Autodesk Inventor part; units mm, degrees
(part 3 of 3)
sketch "Sketch1 outline for Extrusion18" plane through (0, 0, 0) normal (1, 0, 0) x (0, 1, 0)
  line L0 (33.007036, -41.557309) -> (32.83808, -40.490169)
  line L1 (32.83808, -40.490169) -> (32.684563, -39.64781)
  line L2 (32.684563, -39.64781) -> (32.342536, -38.633206)
  line L3 (32.342536, -38.633206) -> (31.917915, -37.441578)
  line L4 (31.917915, -37.441578) -> (31.333308, -36.42555)
  line L5 (31.333308, -36.42555) -> (30.795289, -35.506434)
  line L6 (30.795289, -35.506434) -> (29.641867, -34.174329)
  line L7 (29.641867, -34.174329) -> (29.315032, -33.800203)
  line L8 (29.315032, -33.800203) -> (27.540481, -32.409054)
  line L9 (27.540481, -32.409054) -> (27.014126, -32.133714)
  line L10 (27.014126, -32.133714) -> (25.524659, -31.369786)
  line L11 (25.524659, -31.369786) -> (24.698398, -31.122197)
  line L12 (24.698398, -31.122197) -> (23.29583, -30.72275)
  line L13 (23.29583, -30.72275) -> (22.602461, -30.632692)
  line L14 (22.602461, -30.632692) -> (21.504026, -30.512373)
  line L15 (21.504026, -30.512373) -> (21.030936, -30.512373)
  line L16 (21.030936, -30.512373) -> (20.906647, -30.514104)
  line L17 (20.906647, -30.514104) -> (20.804876, -30.516691)
  line L18 (20.804876, -30.516691) -> (20.202896, -30.530407)
  line L19 (20.202896, -30.530407) -> (18.407116, -30.815395)
  line L20 (18.407116, -30.815395) -> (16.184616, -31.565203)
  line L21 (16.184616, -31.565203) -> (14.183096, -32.714553)
  line L22 (14.183096, -32.714553) -> (12.450816, -34.213661)
  line L23 (12.450816, -34.213661) -> (11.036036, -36.015029)
  line L24 (11.036036, -36.015029) -> (9.984476, -38.066841)
  line L25 (9.984476, -38.066841) -> (9.346936, -40.324139)
  line L26 (9.346936, -40.324139) -> (9.146306, -42.133114)
  line L27 (9.146306, -42.133114) -> (9.164056, -42.734345)
  line L28 (9.164056, -42.734345) -> (9.174216, -43.325403)
  line L29 (9.174216, -43.325403) -> (9.453616, -45.097561)
  line L30 (9.453616, -45.097561) -> (9.822098, -46.206473)
  line L31 (9.822098, -46.206473) -> (10.19878, -47.320103)
  line L32 (10.19878, -47.320103) -> (10.628979, -48.084172)
  line L33 (10.628979, -48.084172) -> (11.336866, -49.317963)
  line L34 (11.336866, -49.317963) -> (11.882186, -49.960017)
  line L35 (11.882186, -49.960017) -> (12.817178, -51.038904)
  line L36 (12.817178, -51.038904) -> (13.54104, -51.62178)
  line L37 (13.54104, -51.62178) -> (14.594831, -52.448813)
  line L38 (14.594831, -52.448813) -> (15.440099, -52.899261)
  line L39 (15.440099, -52.899261) -> (16.628337, -53.507219)
  line L40 (16.628337, -53.507219) -> (17.574428, -53.796043)
  line L41 (17.574428, -53.796043) -> (18.877281, -54.167378)
  line L42 (18.877281, -54.167378) -> (19.560515, -54.257796)
  line L43 (19.560515, -54.257796) -> (20.689085, -54.381464)
  line L44 (20.689085, -54.381464) -> (21.150316, -54.381464)
  line L45 (21.150316, -54.381464) -> (21.356056, -54.377324)
  line L46 (21.356056, -54.377324) -> (21.378916, -54.377324)
  line L47 (21.378916, -54.377324) -> (21.979406, -54.361994)
  line L48 (21.979406, -54.361994) -> (22.13415, -54.337482)
  line L49 (22.13415, -54.337482) -> (24.575291, -53.808384)
  line L50 (24.575291, -53.808384) -> (25.423153, -53.522407)
  line L51 (25.423153, -53.522407) -> (27.202918, -52.636602)
  line L52 (27.202918, -52.636602) -> (27.998156, -52.179361)
  line L53 (27.998156, -52.179361) -> (29.730436, -50.679973)
  line L54 (29.730436, -50.679973) -> (31.145216, -48.878859)
  line L55 (31.145216, -48.878859) -> (32.196776, -46.825777)
  line L56 (32.196776, -46.825777) -> (32.836856, -44.569749)
  line L57 (32.836856, -44.569749) -> (33.034976, -42.760507)
  line L58 (33.034976, -42.760507) -> (33.022276, -42.159543)
  line L59 (33.022276, -42.159543) -> (33.007036, -41.557309)
  line L60 (-22.169384, -48.611651) -> (-23.518124, -50.252745)
  line L61 (-23.518124, -50.252745) -> (-24.111863, -51.312447)
  line L62 (-24.111863, -51.312447) -> (-24.588154, -52.192295)
  line L63 (-24.588154, -52.192295) -> (-24.905044, -53.119435)
  line L64 (-24.905044, -53.119435) -> (-25.301336, -54.389917)
  line L65 (-25.301336, -54.389917) -> (-25.419783, -55.059031)
  line L66 (-25.419783, -55.059031) -> (-25.56963, -56.17919)
  line L67 (-25.56963, -56.17919) -> (-25.578064, -56.345164)
  line L68 (-25.578064, -56.345164) -> (-25.593304, -56.661836)
  line L69 (-25.593304, -56.661836) -> (-25.593304, -57.024666)
  line L70 (-25.593304, -57.024666) -> (-25.521621, -58.095078)
  line L71 (-25.521621, -58.095078) -> (-25.430368, -58.777249)
  line L72 (-25.430368, -58.777249) -> (-25.204455, -59.836085)
  line L73 (-25.204455, -59.836085) -> (-24.794771, -61.149472)
  line L74 (-24.794771, -61.149472) -> (-24.482688, -61.917917)
  line L75 (-24.482688, -61.917917) -> (-23.833695, -63.116856)
  line L76 (-23.833695, -63.116856) -> (-23.403552, -63.814127)
  line L77 (-23.403552, -63.814127) -> (-22.425656, -64.997007)
  line L78 (-22.425656, -64.997007) -> (-22.021991, -65.457083)
  line L79 (-22.021991, -65.457083) -> (-20.383214, -66.812521)
  line L80 (-20.383214, -66.812521) -> (-19.879408, -67.099838)
  line L81 (-19.879408, -67.099838) -> (-18.440429, -67.879534)
  line L82 (-18.440429, -67.879534) -> (-18.074437, -68.024885)
  line L83 (-18.074437, -68.024885) -> (-16.530305, -68.504563)
  line L84 (-16.530305, -68.504563) -> (-15.016744, -68.589031)
  line L85 (-15.016744, -68.589031) -> (-14.849104, -68.58489)
  line L86 (-14.849104, -68.58489) -> (-14.452864, -68.571098)
  line L87 (-14.452864, -68.571098) -> (-10.625084, -68.415371)
  line L88 (-10.625084, -68.415371) -> (-10.477781, -68.408219)
  line L89 (-10.477781, -68.408219) -> (-9.069068, -67.970607)
  line L90 (-9.069068, -67.970607) -> (-6.901029, -66.782518)
  line L91 (-6.901029, -66.782518) -> (-6.724497, -66.636927)
  line L92 (-6.724497, -66.636927) -> (-4.410069, -64.414728)
  line L93 (-4.410069, -64.414728) -> (-4.038829, -63.964888)
  line L94 (-4.038829, -63.964888) -> (-2.494622, -61.063215)
  line L95 (-2.494622, -61.063215) -> (-2.230518, -60.213444)
  line L96 (-2.230518, -60.213444) -> (-1.848254, -58.490356)
  line L97 (-1.848254, -58.490356) -> (-1.722384, -57.559208)
  line L98 (-1.722384, -57.559208) -> (-1.722384, -56.356162)
  line L99 (-1.722384, -56.356162) -> (-1.79223, -55.839475)
  line L100 (-1.79223, -55.839475) -> (-1.982369, -54.500406)
  line L101 (-1.982369, -54.500406) -> (-2.17304, -53.8869)
  line L102 (-2.17304, -53.8869) -> (-2.717481, -52.211101)
  line L103 (-2.717481, -52.211101) -> (-3.113204, -51.481774)
  line L104 (-3.113204, -51.481774) -> (-3.865434, -50.160677)
  line L105 (-3.865434, -50.160677) -> (-4.4666, -49.432156)
  line L106 (-4.4666, -49.432156) -> (-5.380475, -48.386819)
  line L107 (-5.380475, -48.386819) -> (-6.157427, -47.746057)
  line L108 (-6.157427, -47.746057) -> (-7.207823, -46.941879)
  line L109 (-7.207823, -46.941879) -> (-8.154694, -46.428219)
  line L110 (-8.154694, -46.428219) -> (-9.292197, -45.87547)
  line L111 (-9.292197, -45.87547) -> (-10.362386, -45.543008)
  line L112 (-10.362386, -45.543008) -> (-11.715458, -45.204164)
  line L113 (-11.715458, -45.204164) -> (-12.392664, -45.113647)
  line L114 (-12.392664, -45.113647) -> (-13.657176, -45.024663)
  line L115 (-13.657176, -45.024663) -> (-14.090958, -45.024663)
  line L116 (-14.090958, -45.024663) -> (-14.451188, -45.049937)
  line L117 (-14.451188, -45.049937) -> (-15.697902, -45.216811)
  line L118 (-15.697902, -45.216811) -> (-16.261766, -45.327388)
  line L119 (-16.261766, -45.327388) -> (-17.578172, -45.736339)
  line L120 (-17.578172, -45.736339) -> (-18.526645, -46.082568)
  line L121 (-18.526645, -46.082568) -> (-19.456689, -46.586467)
  line L122 (-19.456689, -46.586467) -> (-20.493311, -47.193856)
  line L123 (-20.493311, -47.193856) -> (-21.065728, -47.667296)
  line L124 (-21.065728, -47.667296) -> (-22.169384, -48.611651)
  line L125 (-52.369984, -60.267051) -> (-49.128944, -61.227526)
  line L126 (-55.415444, -58.665759) -> (-52.369984, -60.267051)
  line L127 (-57.536344, -57.046585) -> (-55.415444, -58.665759)
  line L128 (-58.158644, -56.423701) -> (-57.536344, -57.046585)
  line L129 (-58.783484, -55.799445) -> (-58.158644, -56.423701)
  line L130 (-60.404004, -53.677275) -> (-58.783484, -55.799445)
  line L131 (-62.004204, -50.634507) -> (-60.404004, -53.677275)
  line L132 (-62.964324, -47.390673) -> (-62.004204, -50.634507)
  line L133 (-63.286904, -44.048795) -> (-62.964324, -47.390673)
  line L134 (-62.964324, -40.705901) -> (-63.286904, -44.048795)
  line L135 (-62.004204, -37.463337) -> (-62.964324, -40.705901)
  line L136 (-60.404004, -34.419147) -> (-62.004204, -37.463337)
  line L137 (-58.783484, -32.297231) -> (-60.404004, -34.419147)
  line L138 (-58.158644, -31.674169) -> (-58.783484, -32.297231)
  line L139 (-57.536344, -31.049837) -> (-58.158644, -31.674169)
  line L140 (-55.415444, -29.430841) -> (-57.536344, -31.049837)
  line L141 (-52.369984, -27.829625) -> (-55.415444, -29.430841)
  line L142 (-49.128944, -26.868997) -> (-52.369984, -27.829625)
  line L143 (-45.786304, -26.547941) -> (-49.128944, -26.868997)
  line L144 (-42.443664, -26.868997) -> (-45.786304, -26.547941)
  line L145 (-39.200084, -27.829625) -> (-42.443664, -26.868997)
  line L146 (-36.157164, -29.430841) -> (-39.200084, -27.829625)
  line L147 (-34.033724, -31.049837) -> (-36.157164, -29.430841)
  line L148 (-33.408884, -31.674169) -> (-34.033724, -31.049837)
  line L149 (-32.789124, -32.297231) -> (-33.408884, -31.674169)
  line L150 (-31.168604, -34.419147) -> (-32.789124, -32.297231)
  line L151 (-29.568404, -37.463337) -> (-31.168604, -34.419147)
  line L152 (-28.605744, -40.705901) -> (-29.568404, -37.463337)
  line L153 (-28.283164, -44.048795) -> (-28.605744, -40.705901)
  line L154 (-28.605744, -47.390673) -> (-28.283164, -44.048795)
  line L155 (-29.568404, -50.634507) -> (-28.605744, -47.390673)
  line L156 (-31.168604, -53.677275) -> (-29.568404, -50.634507)
  line L157 (-32.789124, -55.799445) -> (-31.168604, -53.677275)
  line L158 (-33.408884, -56.423701) -> (-32.789124, -55.799445)
  line L159 (-34.033724, -57.046585) -> (-33.408884, -56.423701)
  line L160 (-36.157164, -58.665759) -> (-34.033724, -57.046585)
  line L161 (-39.200084, -60.267051) -> (-36.157164, -58.665759)
  line L162 (-42.443664, -61.227526) -> (-39.200084, -60.267051)
  line L163 (-45.786304, -61.548633) -> (-42.443664, -61.227526)
  line L164 (-49.128944, -61.227526) -> (-45.786304, -61.548633)
  line L165 (-59.479444, 24.131155) -> (-60.083964, 21.865475)
  line L166 (-60.083964, 21.865475) -> (-60.199445, 20.635684)
  line L167 (-60.199445, 20.635684) -> (-60.235804, 19.618519)
  line L168 (-60.235804, 19.618519) -> (-60.228744, 19.451205)
  line L169 (-60.228744, 19.451205) -> (-60.205884, 18.851765)
  line L170 (-60.205884, 18.851765) -> (-59.895339, 17.084166)
  line L171 (-59.895339, 17.084166) -> (-59.690576, 16.492921)
  line L172 (-59.690576, 16.492921) -> (-59.126949, 14.900308)
  line L173 (-59.126949, 14.900308) -> (-58.65977, 14.095394)
  line L174 (-58.65977, 14.095394) -> (-57.971801, 12.941087)
  line L175 (-57.971801, 12.941087) -> (-57.323583, 12.191296)
  line L176 (-57.323583, 12.191296) -> (-56.476925, 11.244335)
  line L177 (-56.476925, 11.244335) -> (-55.678233, 10.610482)
  line L178 (-55.678233, 10.610482) -> (-54.690294, 9.860171)
  line L179 (-54.690294, 9.860171) -> (-53.784254, 9.384239)
  line L180 (-53.784254, 9.384239) -> (-52.659665, 8.831052)
  line L181 (-52.659665, 8.831052) -> (-51.657409, 8.529209)
  line L182 (-51.657409, 8.529209) -> (-50.388844, 8.190593)
  line L183 (-50.388844, 8.190593) -> (-49.709686, 8.101058)
  line L184 (-49.709686, 8.101058) -> (-48.575756, 7.994027)
  line L185 (-48.575756, 7.994027) -> (-48.224704, 7.994027)
  line L186 (-48.224704, 7.994027) -> (-47.958004, 7.999615)
  line L187 (-47.958004, 7.999615) -> (-47.938503, 7.999615)
  line L188 (-47.938503, 7.999615) -> (-47.828464, 8.003933)
  line L189 (-47.828464, 8.003933) -> (-47.350022, 8.023598)
  line L190 (-47.350022, 8.023598) -> (-46.652701, 8.12955)
  line L191 (-46.652701, 8.12955) -> (-45.680707, 8.299855)
  line L192 (-45.680707, 8.299855) -> (-44.809198, 8.564772)
  line L193 (-44.809198, 8.564772) -> (-43.526766, 9.019144)
  line L194 (-43.526766, 9.019144) -> (-42.720858, 9.425909)
  line L195 (-42.720858, 9.425909) -> (-41.579317, 10.105711)
  line L196 (-41.579317, 10.105711) -> (-40.934583, 10.582054)
  line L197 (-40.934583, 10.582054) -> (-39.793143, 11.604587)
  line L198 (-39.793143, 11.604587) -> (-39.40199, 12.011768)
  line L199 (-39.40199, 12.011768) -> (-38.289337, 13.473296)
  line L200 (-38.289337, 13.473296) -> (-38.109165, 13.74007)
  line L201 (-38.109165, 13.74007) -> (-37.16308, 15.662676)
  line L202 (-37.16308, 15.662676) -> (-37.127948, 15.741932)
  line L203 (-37.127948, 15.741932) -> (-36.528004, 17.991721)
  line L204 (-36.528004, 17.991721) -> (-36.407377, 19.257413)
  line L205 (-36.407377, 19.257413) -> (-36.383619, 20.472644)
  line L206 (-36.383619, 20.472644) -> (-36.384985, 20.504957)
  line L207 (-36.384985, 20.504957) -> (-36.715964, 22.778859)
  line L208 (-36.715964, 22.778859) -> (-36.898866, 23.305176)
  line L209 (-36.898866, 23.305176) -> (-37.482851, 24.950917)
  line L210 (-37.482851, 24.950917) -> (-37.922645, 25.712215)
  line L211 (-37.922645, 25.712215) -> (-38.623993, 26.888971)
  line L212 (-38.623993, 26.888971) -> (-39.285921, 27.663664)
  line L213 (-39.285921, 27.663664) -> (-40.093943, 28.56811)
  line L214 (-40.093943, 28.56811) -> (-40.939105, 29.251808)
  line L215 (-40.939105, 29.251808) -> (-41.847578, 29.942526)
  line L216 (-41.847578, 29.942526) -> (-42.823468, 30.47202)
  line L217 (-42.823468, 30.47202) -> (-43.908, 31.00537)
  line L218 (-43.908, 31.00537) -> (-44.404458, 31.181517)
  line L219 (-44.404458, 31.181517) -> (-46.370504, 31.705943)
  line L220 (-46.370504, 31.705943) -> (-48.181524, 31.876885)
  line L221 (-48.181524, 31.876885) -> (-48.780964, 31.851993)
  line L222 (-48.780964, 31.851993) -> (-49.380404, 31.828625)
  line L223 (-49.380404, 31.828625) -> (-51.173644, 31.514427)
  line L224 (-51.173644, 31.514427) -> (-53.383444, 30.730583)
  line L225 (-53.383444, 30.730583) -> (-55.367184, 29.550753)
  line L226 (-55.367184, 29.550753) -> (-57.074064, 28.023959)
  line L227 (-57.074064, 28.023959) -> (-58.458364, 26.200747)
  line L228 (-58.458364, 26.200747) -> (-59.479444, 24.131155)
  line L229 (-9.649724, 33.651837) -> (-11.958584, 33.632533)
  line L230 (-7.345944, 33.213687) -> (-9.649724, 33.651837)
  line L231 (-5.639064, 32.579703) -> (-7.345944, 33.213687)
  line L232 (-5.105664, 32.297255) -> (-5.639064, 32.579703)
  line L233 (-4.577344, 32.016077) -> (-5.105664, 32.297255)
  line L234 (-3.099064, 30.953341) -> (-4.577344, 32.016077)
  line L235 (-1.448064, 29.287609) -> (-3.099064, 30.953341)
  line L236 (-0.175524, 27.363813) -> (-1.448064, 29.287609)
  line L237 (0.700776, 25.247231) -> (-0.175524, 27.363813)
  line L238 (1.111089, 23.222486) -> (0.700776, 25.247231)
  line L239 (1.165157, 21.742405) -> (1.111089, 23.222486)
  line L240 (1.172107, 20.840768) -> (1.165157, 21.742405)
  line L241 (0.899345, 19.25247) -> (1.172107, 20.840768)
  line L242 (0.747134, 18.449733) -> (0.899345, 19.25247)
  line L243 (0.310087, 17.242941) -> (0.747134, 18.449733)
  line L244 (0.104117, 16.687319) -> (0.310087, 17.242941)
  line L245 (-0.178064, 16.154793) -> (0.104117, 16.687319)
  line L246 (-0.468312, 15.612618) -> (-0.178064, 16.154793)
  line L247 (-0.902103, 15.008527) -> (-0.468312, 15.612618)
  line L248 (-1.849187, 13.821679) -> (-0.902103, 15.008527)
  line L249 (-2.505593, 13.172266) -> (-1.849187, 13.821679)
  line L250 (-4.28973, 11.767595) -> (-2.505593, 13.172266)
  line L251 (-4.848146, 11.398244) -> (-4.28973, 11.767595)
  line L252 (-7.446953, 10.303356) -> (-4.848146, 11.398244)
  line L253 (-8.75938, 10.036862) -> (-7.446953, 10.303356)
  line L254 (-9.575058, 9.890829) -> (-8.75938, 10.036862)
  line L255 (-11.778244, 9.872611) -> (-9.575058, 9.890829)
  line L256 (-12.609908, 10.030609) -> (-11.778244, 9.872611)
  line L257 (-14.415298, 10.433739) -> (-12.609908, 10.030609)
  line L258 (-14.788027, 10.572332) -> (-14.415298, 10.433739)
  line L259 (-17.365174, 11.877773) -> (-14.788027, 10.572332)
  line L260 (-18.328904, 12.570599) -> (-17.365174, 11.877773)
  line L261 (-19.365663, 13.616768) -> (-18.328904, 12.570599)
  line L262 (-20.470124, 15.029065) -> (-19.365663, 13.616768)
  line L263 (-21.961104, 18.293727) -> (-20.470124, 15.029065)
  line L264 (-22.568164, 21.832455) -> (-21.961104, 18.293727)
  line L265 (-22.450919, 23.631804) -> (-22.568164, 21.832455)
  line L266 (-22.166844, 25.130137) -> (-22.450919, 23.631804)
  line L267 (-21.72057, 26.328829) -> (-22.166844, 25.130137)
  line L268 (-21.059404, 27.712555) -> (-21.72057, 26.328829)
  line L269 (-19.675191, 29.606141) -> (-21.059404, 27.712555)
  line L270 (-18.975433, 30.299284) -> (-19.675191, 29.606141)
  line L271 (-17.882197, 31.264757) -> (-18.975433, 30.299284)
  line L272 (-16.576816, 32.129378) -> (-17.882197, 31.264757)
  line L273 (-16.244236, 32.331452) -> (-16.576816, 32.129378)
  line L274 (-14.201404, 33.174825) -> (-16.244236, 32.331452)
  line L275 (-11.958584, 33.632533) -> (-14.201404, 33.174825)
  line L276 (23.746196, -15.218779) -> (24.254196, -14.903311)
  line L277 (23.255976, -15.519261) -> (23.746196, -15.218779)
  line L278 (21.082473, -16.40026) -> (23.255976, -15.519261)
  line L279 (19.905491, -16.703853) -> (21.082473, -16.40026)
  line L280 (18.941227, -16.880243) -> (19.905491, -16.703853)
  line L281 (16.994876, -16.988397) -> (18.941227, -16.880243)
  line L282 (15.34623, -16.760947) -> (16.994876, -16.988397)
  line L283 (14.597597, -16.631577) -> (15.34623, -16.760947)
  line L284 (14.035431, -16.440388) -> (14.597597, -16.631577)
  line L285 (11.968166, -15.599136) -> (14.035431, -16.440388)
  line L286 (11.229638, -15.175538) -> (11.968166, -15.599136)
  line L287 (9.490883, -13.860947) -> (11.229638, -15.175538)
  line L288 (8.941532, -13.382981) -> (9.490883, -13.860947)
  line L289 (7.614367, -11.801495) -> (8.941532, -13.382981)
  line L290 (7.322556, -11.331563) -> (7.614367, -11.801495)
  line L291 (7.165811, -11.076474) -> (7.322556, -11.331563)
  line L292 (7.109196, -10.977487) -> (7.165811, -11.076474)
  line L293 (6.963602, -10.720747) -> (7.109196, -10.977487)
  line L294 (6.517957, -9.725576) -> (6.963602, -10.720747)
  line L295 (6.225389, -9.010022) -> (6.517957, -9.725576)
  line L296 (5.995587, -8.120458) -> (6.225389, -9.010022)
  line L297 (5.664674, -6.668788) -> (5.995587, -8.120458)
  line L298 (5.656568, -6.521727) -> (5.664674, -6.668788)
  line L299 (5.580116, -4.420731) -> (5.656568, -6.521727)
  line L300 (5.910316, -2.222869) -> (5.580116, -4.420731)
  line L301 (6.636756, -0.120003) -> (5.910316, -2.222869)
  line L302 (7.744196, 1.821827) -> (6.636756, -0.120003)
  line L303 (8.809351, 3.070527) -> (7.744196, 1.821827)
  line L304 (9.246444, 3.57178) -> (8.809351, 3.070527)
  line L305 (9.815194, 4.052564) -> (9.246444, 3.57178)
  line L306 (10.647556, 4.73483) -> (9.815194, 4.052564)
  line L307 (11.033496, 4.980063) -> (10.647556, 4.73483)
  line L308 (11.165512, 5.065335) -> (11.033496, 4.980063)
  line L309 (11.208756, 5.092077) -> (11.165512, 5.065335)
  line L310 (11.589468, 5.325969) -> (11.208756, 5.092077)
  line L311 (13.830183, 6.264269) -> (11.589468, 5.325969)
  line L312 (14.964707, 6.556783) -> (13.830183, 6.264269)
  line L313 (16.016046, 6.754612) -> (14.964707, 6.556783)
  line L314 (17.957536, 6.862711) -> (16.016046, 6.754612)
  line L315 (19.962259, 6.58636) -> (17.957536, 6.862711)
  line L316 (20.621162, 6.415469) -> (19.962259, 6.58636)
  line L317 (22.392376, 5.812675) -> (20.621162, 6.415469)
  line L318 (24.396436, 4.666119) -> (22.392376, 5.812675)
  line L319 (26.164276, 3.124339) -> (24.396436, 4.666119)
  line L320 (26.657089, 2.522869) -> (26.164276, 3.124339)
  line L321 (28.23602, 0.046481) -> (26.657089, 2.522869)
  line L322 (28.689036, -0.968617) -> (28.23602, 0.046481)
  line L323 (29.275776, -3.240901) -> (28.689036, -0.968617)
  line L324 (29.402776, -5.543919) -> (29.275776, -3.240901)
  line L325 (29.087816, -7.811885) -> (29.402776, -5.543919)
  line L326 (28.443584, -9.707927) -> (29.087816, -7.811885)
  line L327 (27.76169, -11.007272) -> (28.443584, -9.707927)
  line L328 (27.305264, -11.802786) -> (27.76169, -11.007272)
  line L329 (26.260434, -13.063339) -> (27.305264, -11.802786)
  line L330 (25.715234, -13.689419) -> (26.260434, -13.063339)
  line L331 (24.776107, -14.47572) -> (25.715234, -13.689419)
  line L332 (24.254196, -14.903311) -> (24.776107, -14.47572)
extrude "Extrusion18" add sketch "Sketch1 outline for Extrusion18" against normal blind 0.25
sketch "Sketch1 outline for Extrusion19" plane through (0, 0, 0) normal (1, 0, 0) x (0, 1, 0)
  line L0 (-45.748204, -44.792152) -> (-39.464718, -51.074948)
  line L1 (-52.03169, -51.074948) -> (-45.748204, -44.792152)
  line L2 (-52.738836, -50.36788) -> (-52.03169, -51.074948)
  line L3 (-46.45535, -44.085084) -> (-52.738836, -50.36788)
  line L4 (-53.343278, -37.197912) -> (-46.45535, -44.085084)
  line L5 (-52.63621, -36.490766) -> (-53.343278, -37.197912)
  line L6 (-45.748204, -43.378016) -> (-52.63621, -36.490766)
  line L7 (-38.860198, -36.490766) -> (-45.748204, -43.378016)
  line L8 (-38.153052, -37.197834) -> (-38.860198, -36.490766)
  line L9 (-45.041058, -44.085084) -> (-38.153052, -37.197834)
  line L10 (-38.75765, -50.367802) -> (-45.041058, -44.085084)
  line L11 (-39.464718, -51.074948) -> (-38.75765, -50.367802)
extrude "Extrusion19" cut sketch "Sketch1 outline for Extrusion19" along normal through all both and the other way through all
body "Solid2"
